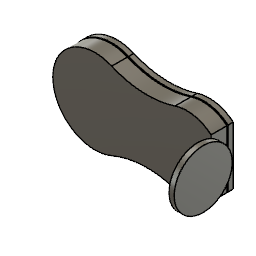
answer (Autodesk Fusion 360 design; units mm, degrees)
part number: 2026-08-05-21-08-28-106
Autodesk Fusion 360 part; units mm, degrees
note: some values were not read from the file. Set by a fixed rule: which sketch regions a step uses.
sketch "Sketch1" plane through (0, 0, 0) normal (1, 0, 0) x (0, 0, -1)
  circle A0 centre (0, 0) radius 27.5
  dimension "d1" = 55
  constraint coincident A0.centre origin
  measures "d1" diameter of A0
extrude "Extrude1" add sketch "Sketch1" along normal blind 5
ref_plane "WorkPlane1" through (0, 0, -27.5) normal (0, 0, 1) x (1, 0, 0)
sketch "Sketch2" plane through (0, 0, -27.5) normal (0, 0, 1) x (1, 0, 0)
  line L0 (0, 0) -> (-150, 0)
  line L1 (0, 0) -> (-23, 0)
  line L2 (-150, 0) -> (-110, 0)
  line L3 (0, 0) -> (0, 27.5)
  circle A0 centre (-23, 0) radius 35.8504
  circle A1 centre (-110, 0) radius 40
  line L4 (0, 27.5) -> (0, -27.5)
  arc A2 (-94.2038, 36.7489) -> (-34.165, 34.0675) centre (-60.6369, 114.8402) ccw
  arc A3 (-34.165, -34.0675) -> (-94.2038, -36.7489) centre (-60.6369, -114.8402) ccw
  point P0 (0, -27.5)
  point P1 (0, 27.5)
  dimension "d6" = 150
  dimension "d7" = 23
  dimension "d8" = 40
  dimension "d9" = 27.5
  dimension "d10" = 85
  constraint coincident L0.start L1.start
  constraint horizontal L0
  constraint parallel L0 L1
  constraint parallel L0 L2
  constraint perpendicular L1 L3
  constraint coincident L1.end A0.centre
  constraint coincident P1 A0
  constraint coincident L0 L2.end
  constraint coincident L0.end A1
  constraint coincident A0 P0
  constraint parallel L3 L4
  constraint coincident A1 A2.start
  constraint coincident A0 A2.end
  constraint tangent A0 A2
  constraint tangent A1 A2
  constraint symmetric L0 A2.end A3.start
  constraint symmetric L0 A2.start A3.end
  constraint symmetric L0 A2 A3
  constraint coincident P0 L4.end
  constraint coincident P1 L3.end
  measures "d6" distance of L0.start L0.end
  measures "d7" distance of L0.start L1.end
  measures "d8" distance of L0.end L2.end
  measures "d9" distance of L0.start L3.end
  measures "d10" radius of A2
extrude "Extrude2" add sketch "Sketch2" along normal blind 15 contours L0 L1 A0 L4 | L0 L1 L3 A0 L4 | L0 A0 A1 A3 | L0 A0 A1 A2 | L0 L2 A1 | L0 L2 A1
sketch "Sketch3" plane through (0, 0, -27.5) normal (0, 0, -1) x (-1, 0, 0)
  arc A0 (34.165, 34.0675) -> (0, 27.5) centre (23, 0) ccw
  line L0 (0, 27.5) -> (0, 0)
  line L1 (0, 0) -> (0, -27.5)
  arc A1 (0, -27.5) -> (34.165, -34.0675) centre (23, 0) ccw
  arc A2 (94.2038, -36.7489) -> (34.165, -34.0675) centre (60.6369, -114.8402) ccw
  arc A3 (94.2038, -36.7489) -> (94.2038, 36.7489) centre (110, 0) ccw
  arc A4 (34.165, 34.0675) -> (94.2038, 36.7489) centre (60.6369, 114.8402) ccw
  arc A5 (95.1911, -34.4521) -> (95.1911, 34.4521) centre (110, 0) ccw
  arc A6 (33.3864, 31.6918) -> (95.1911, 34.4521) centre (60.6369, 114.8402) ccw
  arc A7 (33.3864, 31.6918) -> (2.5, 26.3059) centre (23, 0) ccw
  line L2 (2.5, 26.3059) -> (2.5, 0)
  line L3 (2.5, 0) -> (2.5, -26.3059)
  arc A8 (2.5, -26.3059) -> (33.3864, -31.6918) centre (23, 0) ccw
  arc A9 (95.1911, -34.4521) -> (33.3864, -31.6918) centre (60.6369, -114.8402) ccw
  dimension "d13" = 2.5
extrude "Extrude3" add sketch "Sketch3" along normal blind 1 contours A5 A6 A7 L2 L3 A8 A9
sketch "Sketch4" plane through (0, 0, -28.5) normal (0, 0, -1) x (-1, 0, 0)
  arc A0 (33.3864, 31.6918) -> (2.5, 26.3059) centre (23, 0) ccw
  line L0 (2.5, 26.3059) -> (2.5, -26.3059)
  arc A1 (2.5, -26.3059) -> (33.3864, -31.6918) centre (23, 0) ccw
  arc A2 (95.1911, -34.4521) -> (33.3864, -31.6918) centre (60.6369, -114.8402) ccw
  arc A3 (95.1911, -34.4521) -> (95.1911, 34.4521) centre (110, 0) ccw
  arc A4 (33.3864, 31.6918) -> (95.1911, 34.4521) centre (60.6369, 114.8402) ccw
  arc A5 (94.2038, -36.7489) -> (94.2038, 36.7489) centre (110, 0) ccw
  arc A6 (34.165, 34.0675) -> (94.2038, 36.7489) centre (60.6369, 114.8402) ccw
  arc A7 (34.165, 34.0675) -> (0, 27.5) centre (23, 0) ccw
  line L1 (0, 27.5) -> (0, -27.5)
  arc A8 (0, -27.5) -> (34.165, -34.0675) centre (23, 0) ccw
  arc A9 (94.2038, -36.7489) -> (34.165, -34.0675) centre (60.6369, -114.8402) ccw
  dimension "d16" = -2.5
extrude "Extrude4" add sketch "Sketch4" along normal blind 5 contours A0 L0 A1 A2 A3 A4 | A5 A6 A7 L1 A8 A9
extrude "Extrude5" add 1 faces at (-110.551, 8.9771, -33.5) along direction (0, 0, -1) blind 6.5 draft -65
sketch "Sketch5" plane through (0, 0, -40) normal (0, 0, -1) x (-1, 0, 0)
  arc A0 (29.8238, 20.8214) -> (99.7085, 23.9425) centre (60.6369, 114.8402) ccw
  arc A1 (29.8238, 20.8214) -> (13.9393, 19.9499) centre (23, 0) ccw
  line L0 (13.9393, 19.9499) -> (13.9393, -19.9499)
  arc A2 (13.9393, -19.9499) -> (29.8238, -20.8214) centre (23, 0) ccw
  arc A3 (99.7085, -23.9425) -> (29.8238, -20.8214) centre (60.6369, -114.8402) ccw
  arc A4 (99.7085, -23.9425) -> (99.7085, 23.9425) centre (110, 0) ccw
  line L1 (150, 0) -> (146, 0)
  circle A5 centre (146, 0) radius 4
  line L2 (146, 4) -> (151, 4)
  line L3 (146, -4) -> (151, -4)
  line L4 (151, 4) -> (151, -4)
  dimension "d21" = 4
  dimension "d22" = 8
  dimension "d23" = 5
  constraint horizontal L1
  constraint coincident L1.end A5.centre
  constraint coincident A5 L2.start
  constraint parallel L1 L2
  constraint coincident A5 L3.start
  constraint horizontal L3
  measures "d21" distance of L1.start L1.end
  measures "d22" diameter of A5
  measures "d23" distance of L3.start L3.end
extrude "Extrude6" cut sketch "Sketch5" against normal blind 6.5 contours A5 | A5 L2 L3 L4
